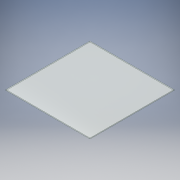
# Autodesk Inventor part: Plate
Saved by Autodesk Inventor 2019 (Build 230136000, 136)
## iProperties
Created: 2019-01-30
Part Number: Plate
Material: Szkło
Document SubType Name: Modeling
Designer: atmat
Density: 2.18 g/cm^3
Appearance: Przezroczyste
Mass: 21.8 g
Surface Area: 204 cm^2
Volume: 10 cm^3
Author: atmat
Autodesk Inventor part; units mm, degrees
ref_plane "YZ Plane" through (0, 0, 0) normal (1, 0, 0) x (0, 1, 0)
ref_plane "XZ Plane" through (0, 0, 0) normal (0, 1, 0) x (-1, 0, 0)
ref_plane "XY Plane" through (0, 0, 0) normal (0, 0, 1) x (1, 0, 0)
sketch "Szkic1" plane through (0, 0, 0) normal (0, 1, 0) x (-1, 0, 0)
  line L0 (50, 50) -> (-50, 50)
  line L1 (-50, 50) -> (-50, -50)
  line L2 (-50, -50) -> (50, -50)
  line L3 (50, -50) -> (50, 50)
  point P0 (0, 0)
  dimension "d0" = 50
  dimension "d1" = 100
  dimension "d2" = 100
  dimension "d3" = 50
  constraints: 8 end point, 2 parallel, 1 horizontal, 1 perpendicular
  measures "d0" distance from line of point (0, 0) L2
  measures "d1" distance of L2.end L0.start
  measures "d2" distance of L1.end L2.end
  measures "d3" distance from line of point (0, 0) L3
extrude "Wyciągnięcie proste1" add sketch "Szkic1" along normal blind 1
